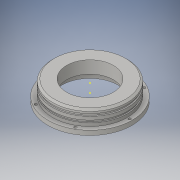
# Autodesk Inventor part: O ring Dome 2
Saved by Autodesk Inventor 2016 (Build 200138000, 138)
## iProperties
Created: 2017-01-20
Part Number: O ring Dome 2
Material: Generic
Document SubType Name: Modeling
Designer: Student
Density: 1 g/cm^3
Appearance: Default
Author: Student
Autodesk Inventor part; units mm, degrees
ref_plane "YZ Plane" through (0, 0, 0) normal (1, 0, 0) x (0, 1, 0)
ref_plane "XZ Plane" through (0, 0, 0) normal (0, 1, 0) x (-1, 0, 0)
ref_plane "XY Plane" through (0, 0, 0) normal (0, 0, 1) x (1, 0, 0)
sketch "Sketch1" plane through (0, 0, 0) normal (0, 1, 0) x (-1, 0, 0)
  circle A0 centre (0, 0) radius 50.8
  dimension "d0" = 101.6
  constraints: 1 centre point, 1 coincident
  measures "d0" diameter of A0
extrude "Extrusion1" add sketch "Sketch1" along normal blind 7.62
sketch "Sketch2" plane through (0, 7.62, 0) normal (0, 1, 0) x (1, 0, 0)
  circle A0 centre (0, 0) radius 49.2125
  circle A1 centre (0, 0) radius 50.8
  dimension "d3" = 98.425
  constraints: 2 centre point, 2 coincident
  measures "d3" diameter of A0
extrude "Extrusion2" cut sketch "Sketch2" against normal blind 3.175
sketch "Sketch3" plane through (0, 7.62, 0) normal (0, 1, 0) x (1, 0, 0)
  circle A0 centre (0, 0) radius 50.9584
  constraints: 1 centre point, 1 coincident
extrude "Extrusion3" add sketch "Sketch3" along normal blind 7.62
sketch "Sketch4" plane through (0, 15.24, 0) normal (0, 1, 0) x (1, 0, 0)
  point P0 (0, 0)
sketch "Sketch5" plane through (0, 15.24, 0) normal (0, 1, 0) x (1, 0, 0)
  circle A0 centre (0, 0) radius 49.2125
  circle A1 centre (0, 0) radius 50.9584
  dimension "d8" = 98.425
  constraints: 2 centre point, 2 coincident
  measures "d8" diameter of A0
extrude "Extrusion4" cut sketch "Sketch5" against normal blind 3.175
sketch "Sketch6" plane through (0, 15.24, 0) normal (0, 1, 0) x (1, 0, 0)
  circle A0 centre (0, 0) radius 50.8
  dimension "d11" = 101.6
  constraints: 1 centre point, 1 coincident
  measures "d11" diameter of A0
extrude "Extrusion5" add sketch "Sketch6" along normal blind 5.08
sketch "Sketch7" plane through (0, 0, 0) normal (0, -1, 0) x (1, 0, 0)
  circle A0 centre (0, 0) radius 57.15
  dimension "d14" = 114.3
  constraints: 1 centre point, 1 coincident
  measures "d14" diameter of A0
extrude "Extrusion6" add sketch "Sketch7" along normal blind 6.096
chamfer "Chamfer1" distance 2.54 angle 45 1 edges at (-50.8, 20.32, 0)
sketch "Sketch8" plane through (0, -6.096, 0) normal (0, -1, 0) x (1, 0, 0)
  circle A0 centre (0, 0) radius 50.8
  circle A1 centre (53.975, 0) radius 1.7526
  circle A2 centre (26.9875, 46.7437) radius 1.7526
  circle A3 centre (-26.9875, 46.7437) radius 1.7526
  circle A4 centre (-53.975, 0) radius 1.7526
  circle A5 centre (-26.9875, -46.7437) radius 1.7526
  circle A6 centre (26.9875, -46.7437) radius 1.7526
  circle A7 centre (46.7437, 26.9875) radius 1.7526
  circle A8 centre (26.9875, 46.7437) radius 1.7526
  circle A9 centre (0, 53.975) radius 1.7526
  circle A10 centre (-26.9875, 46.7437) radius 1.7526
  circle A11 centre (-46.7437, 26.9875) radius 1.7526
  circle A12 centre (-53.975, 0) radius 1.7526
  circle A13 centre (-46.7437, -26.9875) radius 1.7526
  circle A14 centre (-26.9875, -46.7437) radius 1.7526
  circle A15 centre (0, -53.975) radius 1.7526
  circle A16 centre (26.9875, -46.7437) radius 1.7526
  circle A17 centre (46.7437, -26.9875) radius 1.7526
  dimension "d20" = 3.5052
  dimension "d21" = 53.975
  dimension "d24" = 360
  dimension "d44" = 360
  constraints: 18 centre point, 3 coincident, 48 other
  measures "d20" diameter of A1
  measures "d21" distance of A0.centre A1.centre
extrude "Extrusion7" cut sketch "Sketch8" against normal blind 6.096 contours A1 | A2 | A3 | A4 | A5 | A6
sketch "Sketch9" plane through (0, -6.096, 0) normal (0, -1, 0) x (1, 0, 0)
  circle A0 centre (0, 0) radius 12.7
  circle A1 centre (0, 0) radius 1.27
  dimension "d28" = 25.4
  dimension "d29" = 2.54
  constraints: 2 centre point, 2 coincident
  measures "d28" diameter of A0
  measures "d29" diameter of A1
extrude "Extrusion8" cut sketch "Sketch9" against normal blind 127 contours A1
sketch "Sketch10" plane through (0, -6.096, 0) normal (0, -1, 0) x (1, 0, 0)
  circle A0 centre (0, 0) radius 1.27 projected
  circle A1 centre (0, 0) radius 38.1
  dimension "d33" = 76.2
  constraints: 1 centre point, 1 coincident
  measures "d33" diameter of A1
extrude "Extrusion9" cut sketch "Sketch10" against normal blind 9.525
sketch "Sketch11" plane through (0, 3.429, 0) normal (0, -1, 0) x (1, 0, 0)
  circle A0 centre (0, 0) radius 12.7
  circle A1 centre (0, 0) radius 1.27
  dimension "d36" = 25.4
  constraints: 2 centre point, 2 coincident
  measures "d36" diameter of A0
extrude "Extrusion10" add sketch "Sketch11" along normal blind 9.525
sketch "Sketch12" plane through (0, -6.096, 0) normal (0, -1, 0) x (1, 0, 0)
  circle A0 centre (0, 0) radius 31.75
  dimension "d39" = 63.5
  constraints: 1 centre point, 1 coincident
  measures "d39" diameter of A0
extrude "Extrusion11" cut sketch "Sketch12" against normal blind 40.64
sketch "Sketch13" plane through (0, 3.429, 0) normal (0, -1, 0) x (1, 0, 0)
  point P0 (0, 0)
sketch "Sketch14" plane through (0, -6.096, 0) normal (0, -1, 0) x (1, 0, 0)
  point P0 (0, 0)
sketch "Sketch15" plane through (0, -6.096, 0) normal (0, -1, 0) x (1, 0, 0)
  circle A0 centre (0, 0) radius 46.99
  circle A1 centre (0, 0) radius 43.815
  dimension "d46" = 93.98
  dimension "d47" = 87.63
  constraints: 2 centre point, 2 coincident
  measures "d46" diameter of A0
  measures "d47" diameter of A1
extrude "Extrusion12" cut sketch "Sketch15" against normal blind 3.175
sketch "Sketch16" plane through (0, -6.096, 0) normal (0, -1, 0) x (1, 0, 0)
  point P0 (0, 0)
body "Solid1"
